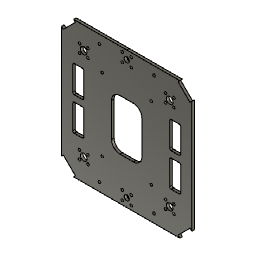
frame base (Autodesk Fusion 360 design; units mm, degrees)
Autodesk Fusion 360 part; units mm, degrees
sketch "Sketch1" plane through (0, 0, 0) normal (0, 1, 0) x (1, 0, 0)
  line L0 (0, -80.6419) -> (154, -80.6419)
  line L1 (33.2319, -142.1916) -> (14.14, -161.2835)
  line L2 (0, -147.1435) -> (19.0919, -128.0516)
  circle A0 centre (21.2132, -140.0682) radius 1.5
  circle A1 centre (26.1614, -142.119) radius 1.5
  circle A2 centre (31.1106, -140.0703) radius 1.5
  circle A3 centre (26.163, -135.1205) radius 4
  circle A4 centre (19.1645, -135.119) radius 1.5
  circle A5 centre (21.2153, -130.1708) radius 1.5
  circle A6 centre (31.1127, -130.1729) radius 1.5
  line L3 (28.9914, -132.2921) -> (33.2341, -128.0495)
  arc A7 (33.11, -142.3135) -> (18.9701, -128.1734) centre (26.163, -135.1205) ccw
  line L4 (77, 0) -> (77, -161.2837)
  line L5 (77, -80.6419) -> (116.5, -80.6419)
  line L6 (116.5, -80.6419) -> (116.5, -130.6419)
  line L7 (116.5, -130.6419) -> (37.5, -130.6419)
  line L8 (37.5, -130.6419) -> (37.5, -30.6419)
  line L9 (37.5, -30.6419) -> (116.5, -30.6419)
  line L10 (116.5, -30.6419) -> (116.5, -80.6419)
  line L11 (95, -80.6419) -> (106, -80.6419)
  line L12 (106, -80.6419) -> (106, -123.5239)
  circle A8 centre (106, -123.5238) radius 1.5
  line L13 (106, -123.5238) -> (48, -123.5238)
  line L14 (48, -123.5238) -> (48, -37.7599)
  line L15 (48, -37.7599) -> (106, -37.7599)
  line L16 (106, -37.7599) -> (106, -80.6419)
  circle A9 centre (48, -123.5238) radius 1.5
  circle A10 centre (48, -37.7599) radius 1.5
  circle A11 centre (106, -37.7599) radius 1.5
  line L17 (9.1913, -9.1915) -> (23.3345, -23.3347)
  line L18 (0, -14.1402) -> (19.0919, -33.2321)
  line L19 (33.2319, -19.0921) -> (14.14, -0.0002)
  circle A12 centre (26.1614, -19.1647) radius 1.5
  circle A13 centre (31.1106, -21.2134) radius 1.5
  circle A14 centre (26.163, -26.1632) radius 4
  circle A15 centre (21.2132, -21.2155) radius 1.5
  circle A16 centre (19.1645, -26.1647) radius 1.5
  circle A17 centre (21.2153, -31.1129) radius 1.5
  arc A18 (18.9701, -33.1103) -> (33.11, -18.9702) centre (26.163, -26.1632) ccw
  line L20 (28.9914, -28.9916) -> (33.2341, -33.2342)
  circle A19 centre (31.1127, -31.1108) radius 1.5
  line L21 (120.7681, -142.1916) -> (139.86, -161.2835)
  line L22 (154, -147.1435) -> (134.9081, -128.0516)
  line L23 (125.0086, -132.2921) -> (120.7659, -128.0495)
  circle A20 centre (127.837, -135.1205) radius 4
  circle A21 centre (122.8894, -140.0703) radius 1.5
  circle A22 centre (127.8386, -142.119) radius 1.5
  arc A23 (135.0299, -128.1734) -> (120.89, -142.3135) centre (127.837, -135.1205) ccw
  circle A24 centre (122.8873, -130.1729) radius 1.5
  circle A25 centre (132.7847, -130.1708) radius 1.5
  circle A26 centre (134.8355, -135.119) radius 1.5
  circle A27 centre (132.7868, -140.0682) radius 1.5
  arc A28 (120.89, -18.9702) -> (135.0299, -33.1103) centre (127.837, -26.1632) ccw
  circle A29 centre (127.837, -26.1632) radius 4
  circle A30 centre (132.7847, -31.1129) radius 1.5
  circle A31 centre (132.7868, -21.2155) radius 1.5
  circle A32 centre (134.8355, -26.1647) radius 1.5
  line L24 (154, -14.1402) -> (134.9081, -33.2321)
  line L25 (120.7681, -19.0921) -> (139.86, -0.0002)
  circle A33 centre (122.8894, -21.2134) radius 1.5
  circle A34 centre (127.8386, -19.1647) radius 1.5
  line L26 (125.0086, -28.9916) -> (120.7659, -33.2342)
  circle A35 centre (122.8873, -31.1108) radius 1.5
  line L27 (139.86, -161.2835) -> (77, -161.2837)
  line L28 (154, -0.0398) -> (154, -0.0002)
  line L29 (154, -14.1402) -> (154, -147.1435)
  line L30 (139.86, -0.0002) -> (14.14, -0.0002)
  line L31 (0, -0.0002) -> (0, 0)
  line L32 (0, -80.6419) -> (0, -147.1435)
  line L33 (0, -80.6419) -> (0, -14.1402)
  line L34 (14.14, -161.2835) -> (77, -161.2837)
  line L35 (77, -161.2837) -> (77, -145.9627)
  line L36 (116.5, -130.6419) -> (116.5001, -161.2836)
  line L37 (134.3209, -44.8918) -> (129.5209, -44.8918)
  line L38 (127.8209, -46.5918) -> (127.8209, -75.1918)
  line L39 (129.5209, -76.8918) -> (139.1209, -76.8918)
  line L40 (140.8209, -75.1918) -> (140.8209, -46.5918)
  line L41 (139.1209, -44.8918) -> (134.3209, -44.8918)
  line L42 (24.4791, -76.8918) -> (14.8791, -76.8918)
  line L43 (13.1791, -75.1918) -> (13.1791, -46.5918)
  line L44 (14.8791, -44.8918) -> (19.6791, -44.8918)
  line L45 (19.6791, -44.8918) -> (24.4791, -44.8918)
  line L46 (26.1791, -46.5918) -> (26.1791, -75.1918)
  line L47 (140.8209, -86.0919) -> (140.8209, -114.6919)
  line L48 (139.1209, -116.3919) -> (134.3209, -116.3919)
  line L49 (134.3209, -116.3919) -> (129.5209, -116.3919)
  line L50 (127.8209, -114.6919) -> (127.8209, -86.0919)
  line L51 (129.5209, -84.3919) -> (139.1209, -84.3919)
  line L52 (26.1791, -114.6919) -> (26.1791, -86.0919)
  line L53 (19.6791, -116.3919) -> (24.4791, -116.3919)
  line L54 (14.8791, -116.3919) -> (19.6791, -116.3919)
  line L55 (13.1791, -86.0919) -> (13.1791, -114.6919)
  line L56 (24.4791, -84.3919) -> (14.8791, -84.3919)
  line L57 (77, -80.6419) -> (95, -80.6419)
  line L58 (95, -80.6419) -> (95, -100.6419)
  line L59 (85, -110.6419) -> (69, -110.6419)
  line L60 (59, -100.6419) -> (59, -60.6419)
  line L61 (69, -50.6419) -> (85, -50.6419)
  line L62 (95, -60.6418) -> (95, -80.6419)
  arc A36 (26.1791, -86.0919) -> (24.4791, -84.3919) centre (24.4791, -86.0919) ccw
  arc A37 (24.4791, -116.3919) -> (26.1791, -114.6919) centre (24.4791, -114.6919) ccw
  arc A38 (13.1791, -114.6919) -> (14.8791, -116.3919) centre (14.8791, -114.6919) ccw
  arc A39 (14.8791, -84.3919) -> (13.1791, -86.0919) centre (14.8791, -86.0919) ccw
  arc A40 (13.1791, -75.1918) -> (14.8791, -76.8918) centre (14.8791, -75.1918) ccw
  arc A41 (24.4791, -76.8918) -> (26.1791, -75.1918) centre (24.4791, -75.1918) ccw
  arc A42 (26.1791, -46.5918) -> (24.4791, -44.8918) centre (24.4791, -46.5918) ccw
  arc A43 (14.8791, -44.8918) -> (13.1791, -46.5918) centre (14.8791, -46.5918) ccw
  arc A44 (129.5209, -44.8918) -> (127.8209, -46.5918) centre (129.5209, -46.5918) ccw
  arc A45 (140.8209, -46.5918) -> (139.1209, -44.8918) centre (139.1209, -46.5918) ccw
  arc A46 (139.1209, -76.8918) -> (140.8209, -75.1918) centre (139.1209, -75.1918) ccw
  arc A47 (127.8209, -75.1918) -> (129.5209, -76.8918) centre (129.5209, -75.1918) ccw
  arc A48 (127.8209, -114.6919) -> (129.5209, -116.3919) centre (129.5209, -114.6919) ccw
  arc A49 (139.1209, -116.3919) -> (140.8209, -114.6919) centre (139.1209, -114.6919) ccw
  arc A50 (140.8209, -86.0919) -> (139.1209, -84.3919) centre (139.1209, -86.0919) ccw
  arc A51 (129.5209, -84.3919) -> (127.8209, -86.0919) centre (129.5209, -86.0919) ccw
  arc A52 (59, -100.6419) -> (69, -110.6419) centre (69, -100.6419) ccw
  arc A53 (85, -110.6419) -> (95, -100.6419) centre (85, -100.6419) ccw
  arc A54 (95, -60.6418) -> (85, -50.6419) centre (85, -60.6418) ccw
  arc A55 (69, -50.6419) -> (59, -60.6419) centre (69, -60.6419) ccw
  line L63 (95, -80.6419) -> (59, -80.6419)
  line L64 (77, -161.2837) -> (77.0001, -141.2837)
  circle A56 centre (77, -151.2837) radius 3
  line L65 (77, -151.2837) -> (97.314, -151.2837) construction
  line L66 (77, -151.2837) -> (95.5921, -151.2837) construction
  circle A57 centre (82.3033, -156.587) radius 1.5
  circle A58 centre (71.6967, -156.587) radius 1.5
  circle A59 centre (71.6967, -145.9804) radius 1.5
  circle A60 centre (82.3034, -145.9804) radius 1.5
  circle A61 centre (77, -10) radius 3
  circle A62 centre (71.6967, -4.6967) radius 1.5
  circle A63 centre (82.3033, -4.6967) radius 1.5
  circle A64 centre (82.3034, -15.3033) radius 1.5
  circle A65 centre (71.6967, -15.3033) radius 1.5
  line L67 (139.86, -161.2835) -> (137.7387, -159.1622)
  line L68 (137.7387, -159.1622) -> (151.8787, -145.0222)
  line L69 (16.2613, -159.1622) -> (2.1213, -145.0222)
  line L70 (14.14, -161.2835) -> (16.2613, -159.1622)
  line L71 (0, -147.1435) -> (19.0919, -128.0516)
  line L72 (33.2319, -19.0921) -> (14.14, -0.0002)
  line L73 (16.2613, -2.1215) -> (2.1213, -16.2615)
  line L74 (0, -14.1402) -> (19.0919, -33.2321)
  line L75 (139.86, -0.0002) -> (137.7387, -2.1215)
  line L76 (137.7387, -2.1215) -> (151.8787, -16.2615)
  line L77 (154, -14.1402) -> (134.9081, -33.2321)
  circle A66 centre (109.276, -151.2837) radius 1.5
  circle A67 centre (44.724, -151.2837) radius 1.5
  circle A68 centre (44.724, -10) radius 1.5
  circle A69 centre (109.276, -10) radius 1.5
  line L78 (134.9081, -128.0516) -> (130.6665, -132.2932)
  line L79 (125.0097, -137.95) -> (120.7681, -142.1916)
  line L80 (144.8087, -152.0922) -> (130.6655, -137.949)
  line L81 (127.8381, -135.1216) -> (127.837, -135.1205)
  line L82 (9.1913, -152.0922) -> (23.3345, -137.949)
  line L83 (26.1619, -135.1216) -> (26.163, -135.1205)
  line L84 (19.0919, -128.0516) -> (23.3335, -132.2932)
  line L85 (28.9903, -137.95) -> (33.2319, -142.1916)
  line L86 (19.0919, -33.2321) -> (23.3335, -28.9905)
  line L87 (28.9903, -23.3337) -> (33.2319, -19.0921)
  line L88 (134.9081, -33.2321) -> (130.6665, -28.9905)
  line L89 (125.0097, -23.3337) -> (120.7681, -19.0921)
  line L90 (144.8087, -9.1915) -> (130.6655, -23.3347)
  line L91 (127.8381, -26.1621) -> (127.837, -26.1632)
  dimension "d1" = 154
  dimension "d57" = 58
  dimension "d65" = 3
  dimension "d66" = 3
  dimension "d67" = 3
  dimension "d68" = 3
  dimension "d89" = 10
  constraint vertical L28
  constraint coincident L31.end origin
  constraint coincident A3.centre A7.centre
  constraint coincident A7.start L1
  constraint coincident A7.end L2
  constraint midpoint L3.end A7
  constraint midpoint L4 L5.start
  constraint perpendicular L4 L5
  constraint perpendicular L0 L6
  constraint perpendicular L6 L7
  constraint perpendicular L7 L8
  constraint perpendicular L8 L9
  constraint perpendicular L9 L10
  constraint perpendicular L4 L11
  constraint perpendicular L5 L12
  constraint coincident A8.centre L13.start
  constraint perpendicular L12 L13
  constraint perpendicular L13 L14
  constraint perpendicular L14 L15
  constraint perpendicular L15 L16
  constraint coincident L13.end L14.start
  constraint coincident L14.end L15.start
  constraint coincident L15.end L16.start
  constraint symmetric L0 L2.end L18.end
  constraint symmetric L0 A7.start A18.end
  constraint symmetric L0 L1.start L19.start
  constraint symmetric L0 A7.end A18.start
  constraint symmetric L0 L1.end L19.end
  constraint symmetric L0 L2.start L18.start
  constraint symmetric L0 L3.end L20.end
  constraint symmetric L0 A0 A15
  constraint symmetric L0 A1 A12
  constraint symmetric L0 A2 A13
  constraint symmetric L0 A3 A14
  constraint symmetric L0 A4 A16
  constraint symmetric L0 A5 A17
  constraint symmetric L0 A6 A19
  constraint symmetric L0 A7 A18
  constraint symmetric L2.end L4 L22.end
  constraint symmetric A7.start L4 A23.end
  constraint symmetric L1.start L4 L21.start
  constraint symmetric A7.end L4 A23.start
  constraint symmetric L1.end L4 L21.end
  constraint symmetric L2.start L4 L22.start
  constraint symmetric L3.end L4 L23.end
  constraint symmetric A3.centre L4 A20.centre
  constraint symmetric A0 L4 A27
  constraint symmetric A1 L4 A22
  constraint symmetric A2 L4 A21
  constraint symmetric A3 L4 A20
  constraint symmetric A4 L4 A26
  constraint symmetric A5 L4 A25
  constraint symmetric A6 L4 A24
  constraint symmetric A7 L4 A23
  constraint symmetric L4 L18.end L24.end
  constraint symmetric L4 A18.start A28.end
  constraint symmetric L4 L20.end L26.end
  constraint symmetric L4 A18.end A28.start
  constraint symmetric L4 L19.start L25.start
  constraint symmetric L4 L19.end L25.end
  constraint symmetric L4 L18.start L24.start
  constraint symmetric L4 L31.start L28.end
  constraint symmetric L4 A12 A34
  constraint symmetric L4 A13 A33
  constraint symmetric L4 A14 A29
  constraint symmetric L4 A15 A31
  constraint symmetric L4 A16 A32
  constraint symmetric L4 A17 A30
  constraint symmetric L4 A18 A28
  constraint symmetric L4 A19 A35
  constraint coincident L0.end L28
  constraint collinear L28 L29
  constraint perpendicular L0 L32
  constraint perpendicular L34 L35
  constraint coincident L27 L36.end
  constraint perpendicular L27 L36
  constraint perpendicular L37 L38
  constraint perpendicular L38 L39
  constraint perpendicular L39 L40
  constraint parallel L11 L57
  constraint perpendicular L5 L58
  constraint perpendicular L58 L59
  constraint perpendicular L59 L60
  constraint perpendicular L60 L61
  constraint perpendicular L61 L62
  constraint tangent L52 A36
  constraint tangent L56 A36
  constraint tangent L52 A37
  constraint tangent L53 A37
  constraint tangent L54 A38
  constraint tangent L55 A38
  constraint tangent L55 A39
  constraint tangent L56 A39
  constraint tangent L42 A40
  constraint tangent L43 A40
  constraint tangent L42 A41
  constraint tangent L46 A41
  constraint tangent L45 A42
  constraint tangent L46 A42
  constraint tangent L43 A43
  constraint tangent L44 A43
  constraint tangent L37 A44
  constraint tangent L38 A44
  constraint tangent L40 A45
  constraint tangent L41 A45
  constraint tangent L39 A46
  constraint tangent L40 A46
  constraint tangent L38 A47
  constraint tangent L39 A47
  constraint tangent L49 A48
  constraint tangent L50 A48
  constraint tangent L47 A49
  constraint tangent L48 A49
  constraint tangent L47 A50
  constraint tangent L51 A50
  constraint tangent L50 A51
  constraint tangent L51 A51
  constraint tangent L59 A52
  constraint tangent L60 A52
  constraint tangent L58 A53
  constraint tangent L59 A53
  constraint equal A52 A53
  constraint tangent L61 A54
  constraint tangent L62 A54
  constraint equal A52 A54
  constraint tangent L60 A55
  constraint tangent L61 A55
  constraint equal A52 A55
  constraint midpoint L60 L63.end
  constraint perpendicular L60 L63
  constraint perpendicular L34 L64
  constraint horizontal L65
  constraint coincident A56.centre L65.start
  constraint horizontal L66
  constraint symmetric L4 A57 A58
  constraint symmetric L63 A56 A61
  constraint symmetric L63 A57 A63
  constraint symmetric L63 A58 A62
  constraint symmetric L63 A59 A65
  constraint symmetric L63 A60 A64
  constraint coincident L22 L68.end
  constraint perpendicular L22 L68
  constraint symmetric L4 L22.end L2.end
  constraint symmetric L4 L21.end L1.end
  constraint symmetric L4 L22.start L2.start
  constraint symmetric L4 L67.end L69.start
  constraint symmetric L4 L68.end L69.end
  constraint symmetric L0 L22.end L24.end
  constraint symmetric L0 L21.end L25.end
  constraint symmetric L0 L22.start L24.start
  constraint symmetric L0 L67.end L75.end
  constraint symmetric L0 L68.end L76.end
  constraint symmetric L0 L69.start L73.start
  constraint symmetric L0 L69.end L73.end
  constraint coincident L68 L80.start
  constraint coincident L69 L82.start
  constraint coincident L73 L17.start
  constraint coincident L76 L90.start
  constraint symmetric L4 A66 A67
  constraint symmetric L63 A66 A69
  constraint symmetric L63 A67 A68
  constraint coincident L81.start L80
  constraint coincident A20 L79.start
  constraint collinear L78 L79
  constraint coincident A20 L80.end
  constraint collinear L80 L81
  constraint coincident A20 L78.end
  constraint coincident A20 L23.start
  constraint coincident A3 L82.end
  constraint collinear L82 L83
  constraint coincident A3 L85.start
  constraint collinear L84 L85
  constraint coincident A3 L84.end
  constraint coincident A3 L3.start
  constraint coincident A14 L86.end
  constraint collinear L86 L87
  constraint coincident A14 L20.start
  constraint coincident A14 L87.start
  constraint coincident A14 L17.end
  constraint coincident A29 L26.start
  constraint coincident A29 L88.end
  constraint coincident L91.start L90
  constraint collinear L88 L89
  constraint coincident A29 L90.end
  constraint collinear L90 L91
  constraint coincident A29 L89.start
  measures "d1" distance of L31.end L28.start
  measures "d57" distance of L14.end L15.end
  measures "d65" diameter of A8
  measures "d66" diameter of A9
  measures "d67" diameter of A10
  measures "d68" diameter of A11
  measures "d89" radius of A52
extrude "Extrude6" add sketch "Sketch1" along normal blind 3 contours L2 A0 A3 A5 A7 L69 L71 L82 L84 | L17 L18 A14 A15 A17 A18 L73 L74 L86 | L1 A0 A2 A3 A7 L69 L82 L85 | L17 L19 A13 A14 A15 A18 L72 L73 L87 | A28 A29 A30 A31 L24 L76 L77 L88 L90 | L22 A20 A23 A25 A27 L68 L78 L80 | A28 A29 A31 L25 A33 L76 L89 L90 | L21 A20 A21 A23 A27 L68 L79 L80 makes body 1 at (12.8321, 0, 148.4243) makes body 2 at (12.8321, 0, 12.8594) makes body 3 at (141.1679, 3, 148.4243) makes body 4 at (141.1679, 3, 12.8594)
extrude "Extrude1" add sketch "Sketch1" along normal blind 3 separate body contours L0 L4 L60 L61 A55 L63 | L0 L4 L13 L14 A9 L59 L60 A52 | L0 L4 L59 L60 A52 L63 | L0 L4 L14 L15 A10 L60 L61 A55 | L0 L4 L5 L57 L61 L62 A54 L63 | L0 L4 L5 L57 L58 L59 A53 L63 | L0 L4 L7 L8 L13 L14 A9 | L0 L4 L8 L9 L14 L15 A10 | L0 L4 L5 L11 L15 L16 A11 L61 L62 A54 | L0 L4 L5 L11 L12 A8 L13 L58 L59 A53 | L0 L1 L2 A7 L4 L7 L8 L32 L34 L35 L64 A56 L70 L71 | L0 L4 L8 L9 L18 L19 A18 L30 L33 A61 L72 L74 | L0 L4 L5 L9 L10 L15 L16 A11 | L0 L4 L5 L6 L7 L12 A8 L13 | L0 L4 L9 L10 A28 L24 L25 L29 L30 A61 L75 L77 | L0 L6 L21 L22 A23 L27 L29 L36 L67 | L4 L7 L27 L35 L36 L64 A56 | L4 A61 | L4 A61 | L2 A0 A3 A5 A7 L69 L71 L82 L84 | L17 L18 A14 A15 A17 A18 L73 L74 L86 | L1 A0 A2 A3 A7 L69 L82 L85 | L17 L19 A13 A14 A15 A18 L72 L73 L87 | A28 A29 A30 A31 L24 L76 L77 L88 L90 | L22 A20 A23 A25 A27 L68 L78 L80 | L4 L35 L64 A56 | L4 L35 L64 A56 | A3 A5 A6 L3 A7 L84 | A14 A17 A18 L20 A19 L86 | A28 A29 A31 L25 A33 L76 L89 L90 | L21 A20 A21 A23 A27 L68 L79 L80 | A2 A3 A6 L3 A7 L85 | A13 A14 A18 L20 A19 L87 | A28 A29 A30 L26 A35 L88 | L23 A20 A23 A24 A25 L78 | A28 A29 A33 L26 A35 L89 | L23 A20 A21 A23 A24 L79 | A1 | A4 | A12 | A16 | A22 | A32 | A34 | L37 L38 L39 L40 L41 A44 A45 A46 A47 | L42 L43 L44 L45 L46 A40 A41 A42 A43 | L47 L48 L49 L50 L51 A48 A49 A50 A51 | L52 L53 L54 L55 L56 A36 A37 A38 A39 | A57 | A58 | A59 | A60 | A62 | A63 | A64 | A65 | A66 | A67 | A68 | A69 makes body 5
extrude "Extrude2" cut sketch "Sketch1" along normal blind 3 contours L37 L38 L39 L40 L41 A44 A45 A46 A47 | L42 L43 L44 L45 L46 A40 A41 A42 A43 | L47 L48 L49 L50 L51 A48 A49 A50 A51 | L52 L53 L54 L55 L56 A36 A37 A38 A39 bodies 5
extrude "Extrude4" cut sketch "Sketch1" along normal blind 3 contours L0 L4 L60 L61 A55 L63 | L0 L4 L59 L60 A52 L63 | L0 L4 L5 L57 L61 L62 A54 L63 | L0 L4 L5 L57 L58 L59 A53 L63 bodies 5
extrude "Extrude5" cut sketch "Sketch1" along normal blind 3 contours L4 A61 | L4 A61 | L4 L35 L64 A56 | L4 L35 L64 A56 | A57 | A58 | A59 | A60 | A62 | A63 | A64 | A65 bodies 5
extrude "Extrude7" cut sketch "Sketch1" along normal blind 3 contours A66 | A67 | A68 | A69 bodies 5
extrude "Extrude8" add sketch "Sketch1" along normal blind 3 contours L2 A0 A3 A5 A7 L69 L71 L82 L84 | L17 L18 A14 A15 A17 A18 L73 L74 L86 | L1 A0 A2 A3 A7 L69 L82 L85 | L17 L19 A13 A14 A15 A18 L72 L73 L87 | A28 A29 A30 A31 L24 L76 L77 L88 L90 | L22 A20 A23 A25 A27 L68 L78 L80 | A28 A29 A31 L25 A33 L76 L89 L90 | L21 A20 A21 A23 A27 L68 L79 L80 | A1 | A4 | A12 | A16 | A22 | A26 | A32 | A34 bodies 1 2 3 4 5
